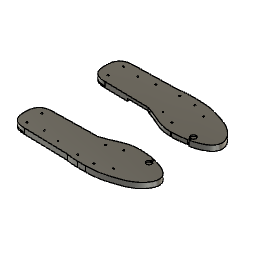
Kids size 4 Insole (Autodesk Fusion 360 design; units mm, degrees)
Autodesk Fusion 360 part; units mm, degrees
note: some values were not read from the file. Chosen so that the rebuilt part matches the saved one: which face or edge a step refers to. Set by a fixed rule: which sketch regions a step uses.
sketch "Sketch2" plane through (0, 0, 0) normal (0, 0, 1) x (1, 0, 0)
  line L0 (0, 0) -> (131.459, 3.2843)
  line L1 (131.459, 3.2843) -> (0, 0.1)
  line L2 (0, 0.1) -> (0, -63.4)
  line L3 (131.459, 3.2843) -> (131.459, -65.9157)
  line L4 (0, -63.4) -> (131.459, -65.9157)
  dimension "d12" = 131.5
  dimension "d13" = 63.5
  dimension "d14" = 69.2
  constraint coincident L0.start origin
  constraint vertical L2
  constraint vertical L3
  measures "d12" distance of L0.start L0.end
  measures "d13" distance of L1.end L2.end
  measures "d14" distance of L0.end L3.end
extrude "Extrude3" add sketch "Sketch2" along normal blind 3 contours L0 L2 L3 L4 makes body 1
fillet "Fillet2" radius 32 tangency weight 1.5916 2 edges at (0, -63.4, 1.5) (0, 0, 1.5) on bodies 1
sketch "Sketch6" plane through (0, 0, 0) normal (0, 0, 1) x (1, 0, 0)
  spline S0 degree 3 poles (0, -31.2105) (0, -25.0639) (0.6991, -19.9859) (3.1095, -12.9138) (4.5302, -10.2219) (8.3444, -5.8662) (10.468, -4.27) (15.3454, -1.7622) (18.03, -0.9116) (24.1411, 0.3806) (27.7349, 0.6929) (31.2008, 0.7795) knots 0 0 0 0 1.843982 1.843982 3.131886 3.131886 4.266621 4.266621 5.428345 5.428345 6.887146 6.887146 6.887146 6.887146
  line L0 (0, -31.2105) -> (0, -32.0065)
  spline S1 degree 3 poles (31.3877, -64.0007) (25.2343, -63.8829) (20.16, -63.0847) (13.1213, -60.5347) (10.451, -59.0604) (6.1653, -55.1613) (4.61, -53.0089) (2.1872, -48.0616) (1.3883, -45.3347) (0.2265, -39.1397) (0, -35.5051) (0, -32.0065) knots 0 0 0 0 1.846381 1.846381 3.135313 3.135313 4.268701 4.268701 5.439843 5.439843 6.910617 6.910617 6.910617 6.910617
  line L1 (31.3877, -64.0007) -> (131.459, -65.9157)
  line L2 (131.459, -65.9157) -> (131.459, 3.2843)
  line L3 (131.459, 3.2843) -> (31.2008, 0.7795)
sketch "Sketch7" plane through (0, 0, 0) normal (0, 0, 1) x (1, 0, 0)
  line L0 (131.459, 3.2843) -> (156.459, 3.2906)
  line L1 (156.459, 3.2906) -> (156.4583, 5.7906)
  line L2 (156.4583, 5.7906) -> (181.4583, 5.7969)
  line L3 (181.4583, 5.7969) -> (206.4583, 5.8032)
  line L4 (206.4583, 5.8032) -> (206.4591, 2.8032)
  line L5 (206.4591, 2.8032) -> (231.4591, 2.8095)
  line L6 (231.4591, 2.8095) -> (231.4609, -4.1905)
  line L7 (231.4609, -4.1905) -> (256.4609, -4.1842)
  line L8 (256.4609, -4.1842) -> (256.4634, -14.1842)
  line L9 (256.4634, -14.1842) -> (281.4634, -14.1779)
  line L10 (281.4634, -14.1779) -> (281.4697, -39.1779)
  line L11 (281.4697, -39.1779) -> (282.4697, -39.1777)
  line L12 (282.4697, -39.1777) -> (282.4728, -51.6776)
  line L13 (282.4728, -51.6776) -> (282.476, -64.1776)
  line L14 (282.476, -64.1776) -> (281.476, -64.1779)
  line L15 (281.476, -64.1779) -> (281.481, -84.1779)
  line L16 (281.481, -84.1779) -> (241.481, -84.188)
  line L17 (241.481, -84.188) -> (241.482, -88.188)
  line L18 (241.482, -88.188) -> (206.482, -88.1968)
  line L19 (206.482, -88.1968) -> (181.482, -88.2031)
  line L20 (181.482, -88.2031) -> (181.4813, -85.2031)
  line L21 (181.4813, -85.2031) -> (156.4813, -85.2094)
  line L22 (156.4813, -85.2094) -> (156.4787, -75.2094)
  line L23 (156.4787, -75.2094) -> (131.4787, -75.2157)
  spline S0 degree 5 poles (131.459, 3.2843) (132.1496, 3.4582) (133.6274, 3.7925) (136.1339, 4.2533) (140.0557, 4.7865) (145.907, 5.3153) (152.6506, 5.6995) (160.1734, 5.9262) (168.2781, 5.9729) (176.6933, 5.8104) (185.1183, 5.4099) (193.2584, 4.7498) (200.8653, 3.8224) (207.7726, 2.6398) (213.9395, 1.2425) (219.4754, -0.2985) (224.5797, -1.9091) (229.489, -3.5365) (234.4262, -5.1721) (239.5391, -6.8834) (244.8868, -8.8023) (250.4574, -11.0844) (256.1762, -13.8773) (261.9178, -17.2853) (267.5158, -21.3344) (272.7732, -25.9844) (277.4708, -31.1438) (281.3773, -36.6842) (284.2586, -42.4544) (285.885, -48.2944) (286.0533, -54.0471) (284.622, -59.5649) (281.5417, -64.7188) (276.8896, -69.4065) (270.8971, -73.5598) (263.8956, -77.1412) (256.2691, -80.1407) (248.4036, -82.5733) (240.6395, -84.4754) (233.2193, -85.9023) (226.2451, -86.925) (219.7173, -87.6165) (213.567, -88.0406) (207.6915, -88.2384) (201.9861, -88.2175) (196.3828, -87.9356) (190.8475, -87.3214) (185.3659, -86.3069) (179.934, -84.8529) (174.5451, -82.9834) (169.1831, -80.7989) (163.8289, -78.4374) (158.4649, -76.0438) (153.0796, -73.7396) (147.6736, -71.5841) (142.2576, -69.5788) (137.9285, -68.0722) (134.6896, -66.981) (132.5348, -66.2682) (131.4585, -65.9154) knots 0 0 0 0 0 0 0.018182 0.036364 0.054545 0.072727 0.090909 0.109091 0.127273 0.145455 0.163636 0.181818 0.2 0.218182 0.236364 0.254545 0.272727 0.290909 0.309091 0.327273 0.345455 0.363636 0.381818 0.4 0.418182 0.436364 0.454545 0.472727 0.490909 0.509091 0.527273 0.545455 0.563636 0.581818 0.6 0.618182 0.636364 0.654545 0.672727 0.690909 0.709091 0.727273 0.745455 0.763636 0.781818 0.8 0.818182 0.836364 0.854545 0.872727 0.890909 0.909091 0.927273 0.945455 0.963636 0.981818 1 1 1 1 1 1
  line L24 (131.459, 3.2843) -> (131.4585, -65.9154)
  line L25 (152.0683, -72.6702) -> (110.8487, -59.1606)
  point P0 (131.459, 3.2843)
  dimension "d41" = 25
  dimension "d42" = 2.5
  dimension "d43" = 25
  dimension "d44" = 25
  dimension "d45" = 3
  dimension "d46" = 25
  dimension "d47" = 7
  dimension "d48" = 25
  dimension "d49" = 10
  dimension "d50" = 25
  dimension "d51" = 25
  dimension "d52" = 1
  dimension "d53" = 12.5
  dimension "d54" = 12.5
  dimension "d55" = 1
  dimension "d56" = 20
  dimension "d57" = 40
  dimension "d58" = 4
  dimension "d59" = 35
  dimension "d60" = 25
  dimension "d63" = 3
  dimension "d64" = 25
  dimension "d65" = 10
  dimension "d66" = 25
  constraint coincident P0 L0.start
  constraint perpendicular L0 L1
  constraint perpendicular L1 L2
  constraint parallel L2 L3
  constraint perpendicular L3 L4
  constraint perpendicular L4 L5
  constraint perpendicular L5 L6
  constraint perpendicular L6 L7
  constraint perpendicular L7 L8
  constraint perpendicular L8 L9
  constraint perpendicular L9 L10
  constraint perpendicular L10 L11
  constraint perpendicular L11 L12
  constraint parallel L12 L13
  constraint perpendicular L13 L14
  constraint perpendicular L14 L15
  constraint perpendicular L15 L16
  constraint perpendicular L16 L17
  constraint perpendicular L17 L18
  constraint parallel L18 L19
  constraint perpendicular L19 L20
  constraint perpendicular L20 L21
  constraint perpendicular L21 L22
  constraint perpendicular L22 L23
  constraint midpoint S0.end L25
  measures "d41" distance of P0 L0.end
  measures "d42" distance of L0.end L1.end
  measures "d43" distance of L1.end L2.end
  measures "d44" distance of L2.end L3.end
  measures "d45" distance of L3.end L4.end
  measures "d46" distance of L4.end L5.end
  measures "d47" distance of L5.end L6.end
  measures "d48" distance of L6.end L7.end
  measures "d49" distance of L7.end L8.end
  measures "d50" distance of L8.end L9.end
  measures "d51" distance of L9.end L10.end
  measures "d52" distance of L10.end L11.end
  measures "d53" distance of L11.end L12.end
  measures "d54" distance of L12.end L13.end
  measures "d55" distance of L13.end L14.end
  measures "d56" distance of L14.end L15.end
  measures "d57" distance of L15.end L16.end
  measures "d58" distance of L16.end L17.end
  measures "d59" distance of L17.end L18.end
  measures "d60" distance of L18.end L19.end
  measures "d63" distance of L19.end L20.end
  measures "d64" distance of L20.end L21.end
  measures "d65" distance of L21.end L22.end
  measures "d66" distance of L22.end L23.end
extrude "Extrude5" add sketch "Sketch7" along normal blind 3 contours L0 L1 S0 | L0 L1 L2 L10 L11 L12 L13 L19 S0 L24 | L10 L11 S0 | L12 L13 S0 bodies 1
hole "Hole2" at (144.8302, -7.2652, 3) direction (0, 0, -1) diameter 3.66 depth 25 tip angle 118 bodies 1
hole "Hole3" at (157.2563, -58.0502, 3) direction (0, 0, -1) diameter 3.66 depth 25 tip angle 118 bodies 1
hole "Hole4" at (23.0004, -13.2082, 3) direction (0, 0, -1) diameter 3.66 depth 25 tip angle 118 bodies 1
hole "Hole5" at (22.3251, -47.9202, 3) direction (0, 0, -1) diameter 3.66 depth 25 tip angle 118 bodies 1
hole "Hole6" at (94.9908, -11.9926, 3) direction (0, 0, -1) diameter 3.66 depth 25 tip angle 118 bodies 1
extrude "Extrude6" add 1 faces at (85.7573, -47.8831, 3) along direction (0, 0, 1) blind 9.25 on bodies 1 bodies 1
hole "Hole8" at (180.2887, -8.2307, 12.25) direction (0, 0, -1) diameter 3.66 depth 25 tip angle 118 bodies 1
hole "Hole9" at (58.9598, -17.4028, 12.25) direction (0, 0, -1) diameter 3.66 depth 25 tip angle 118 bodies 1
hole "Hole10" at (212.5454, -20.8108, 12.25) direction (0, 0, -1) diameter 3.66 depth 25 tip angle 118 bodies 1
hole "Hole12" at (188.1637, -68.6508, 0) direction (0, 0, 1) diameter 3.66 depth 15 tip angle 118 bodies 1
hole "Hole7" at (241.4162, -72.7282, 12.25) direction (0, 0, -1) diameter 12.2 depth 3 tip angle 180 bodies 1
sketch "Sketch8" plane through (0, 0, 12.25) normal (0, 0, 1) x (1, 0, 0)
  line L0 (242.7662, -72.7282) -> (240.0662, -72.7282)
  line L1 (240.0662, -72.7282) -> (240.0662, -84.5002)
  line L2 (240.0662, -84.5002) -> (242.7662, -84.5002)
  line L3 (242.7662, -84.5002) -> (242.7662, -72.7282)
  circle A0 centre (94.9908, -11.9926) radius 1.83
  circle A1 centre (22.3251, -47.9202) radius 1.83
  circle A2 centre (23.0004, -13.2082) radius 1.83
  circle A3 centre (157.2563, -58.0502) radius 1.83
  circle A4 centre (144.8302, -7.2652) radius 1.83
  spline S0 degree 3 poles (31.2008, 0.7795) (27.7349, 0.6929) (24.1411, 0.3806) (18.03, -0.9116) (15.3454, -1.7622) (10.468, -4.27) (8.3444, -5.8662) (4.5302, -10.2219) (3.1095, -12.9138) (0.6991, -19.9859) (0, -25.0639) (0, -31.2105) knots -6.887146 -6.887146 -6.887146 -6.887146 -5.428345 -5.428345 -4.266621 -4.266621 -3.131886 -3.131886 -1.843982 -1.843982 0 0 0 0
  line L4 (0, -31.2105) -> (0, -32.0065)
  spline S1 degree 3 poles (0, -32.0065) (0, -35.5051) (0.2265, -39.1397) (1.3883, -45.3347) (2.1872, -48.0616) (4.61, -53.0089) (6.1653, -55.1613) (10.451, -59.0604) (13.1213, -60.5347) (20.16, -63.0847) (25.2343, -63.8829) (31.3877, -64.0007) knots -6.910617 -6.910617 -6.910617 -6.910617 -5.439843 -5.439843 -4.268701 -4.268701 -3.135313 -3.135313 -1.846381 -1.846381 0 0 0 0
  line L5 (31.3877, -64.0007) -> (131.459, -65.9157)
  spline S2 degree 5 poles (131.459, -65.9156) (132.5352, -66.2683) (134.6899, -66.9811) (137.9287, -68.0722) (142.2577, -69.5788) (147.6736, -71.5841) (153.0796, -73.7396) (158.4649, -76.0438) (163.8289, -78.4374) (169.1831, -80.7989) (174.5451, -82.9834) (179.934, -84.8529) (185.3659, -86.3069) (190.8475, -87.3214) (195.8051, -87.8715) (199.6969, -88.0977) (202.4992, -88.175) (204.1845, -88.1939) (204.7313, -88.1972) knots -0.999998 -0.999998 -0.999998 -0.999998 -0.999998 -0.999998 -0.981818 -0.963636 -0.945455 -0.927273 -0.909091 -0.890909 -0.872727 -0.854545 -0.836364 -0.818182 -0.8 -0.781818 -0.763636 -0.754941 -0.754941 -0.754941 -0.754941 -0.754941 -0.754941
  line L6 (204.7313, -88.1972) -> (206.482, -88.1968)
  spline S3 degree 5 poles (206.482, -88.1968) (206.7317, -88.1952) (208.1358, -88.183) (210.716, -88.1299) (214.5305, -87.9742) (219.7173, -87.6165) (226.2451, -86.925) (233.2193, -85.9023) (240.6395, -84.4754) (248.4036, -82.5733) (256.2691, -80.1407) (263.8956, -77.1412) (270.8971, -73.5598) (276.8896, -69.4065) (281.5417, -64.7188) (284.622, -59.5649) (286.0533, -54.0471) (285.885, -48.2944) (284.2586, -42.4544) (281.3773, -36.6842) (277.4708, -31.1438) (272.7732, -25.9844) (267.5158, -21.3344) (261.9178, -17.2853) (256.1762, -13.8773) (250.4574, -11.0844) (244.8868, -8.8023) (239.5391, -6.8834) (234.4262, -5.1721) (229.489, -3.5365) (224.5797, -1.9091) (219.4754, -0.2985) (213.9395, 1.2425) (207.7726, 2.6398) (200.8653, 3.8224) (193.2584, 4.7498) (186.4723, 5.3001) (181.1712, 5.5881) (177.5263, 5.7278) (175.5655, 5.7871) (175.283, 5.7954) knots -0.749394 -0.749394 -0.749394 -0.749394 -0.749394 -0.749394 -0.745455 -0.727273 -0.709091 -0.690909 -0.672727 -0.654545 -0.636364 -0.618182 -0.6 -0.581818 -0.563636 -0.545455 -0.527273 -0.509091 -0.490909 -0.472727 -0.454545 -0.436364 -0.418182 -0.4 -0.381818 -0.363636 -0.345455 -0.327273 -0.309091 -0.290909 -0.272727 -0.254545 -0.236364 -0.218182 -0.2 -0.181818 -0.163636 -0.145455 -0.127273 -0.124212 -0.124212 -0.124212 -0.124212 -0.124212 -0.124212
  line L7 (175.283, 5.7954) -> (156.4583, 5.7906)
  spline S4 degree 5 poles (156.4583, 5.7906) (155.7183, 5.7686) (153.5076, 5.6957) (149.9506, 5.5432) (145.3158, 5.2618) (140.0557, 4.7865) (136.1339, 4.2533) (133.6274, 3.7925) (132.1496, 3.4582) (131.459, 3.2843) knots -0.081724 -0.081724 -0.081724 -0.081724 -0.081724 -0.081724 -0.072727 -0.054545 -0.036364 -0.018182 0 0 0 0 0 0
  line L8 (131.459, 3.2843) -> (31.2008, 0.7795)
  circle A5 centre (212.5454, -20.8108) radius 1.83
  circle A6 centre (58.9598, -17.4028) radius 1.83
  circle A7 centre (180.2887, -8.2307) radius 1.83
  circle A8 centre (188.1637, -68.6508) radius 1.83
  circle A9 centre (241.4162, -72.7282) radius 6.1
  point P0 (241.4162, -72.7282)
  point P1 (241.4162, -72.7282)
  point P2 (241.4162, -72.7282)
  dimension "d91" = 2.7
  constraint horizontal L0
  constraint vertical L1
  constraint horizontal L2
  constraint vertical L3
  constraint midpoint L0 P2
  constraint coincident P2 P1
  constraint coincident L1.end S3
  measures "d91" distance of L0.start L0.end
extrude "Extrude7" cut sketch "Sketch8" against normal blind 2.7 contours L1 L3 S3 A9 bodies 1
sketch "Sketch9" plane through (0, 0, 0) normal (0, 0, 1) x (1, 0, 0)
  line L0 (83.1727, -66.3805) -> (151.6727, -66.3805)
  line L1 (151.6727, -66.3805) -> (151.6727, -18.3805)
  line L2 (151.6727, -18.3805) -> (83.1727, -18.3805)
  line L3 (83.1727, -18.3805) -> (83.1727, -66.3805)
  dimension "d94" = 68.5
  dimension "d214" = 48
  constraint horizontal L0
  constraint vertical L1
  constraint horizontal L2
  constraint vertical L3
  measures "d94" distance of L0.start L0.end
  measures "d214" distance of L0.start L2.end
extrude "Extrude8" cut sketch "Sketch9" along normal blind 5.5 bodies 1
sketch "Sketch21" plane through (0, 0, 0) normal (0, 0, -1) x (1, 0, 0)
  line L0 (83.1727, 18.3805) -> (83.1727, 64.9916)
  line L1 (83.1727, 64.9916) -> (31.3877, 64.0007)
  spline S0 degree 3 poles (0, 32.0065) (0, 38.1611) (0.7009, 43.2497) (3.1158, 50.3359) (4.5388, 53.034) (8.3551, 57.3935) (10.4774, 58.9897) (15.3774, 61.5066) (18.0886, 62.3576) (24.2602, 63.6377) (27.8898, 63.9337) (31.3877, 64.0007) knots 0 0 0 0 1.846381 1.846381 3.135313 3.135313 4.268701 4.268701 5.439843 5.439843 6.910617 6.910617 6.910617 6.910617
  line L2 (0, 32.0065) -> (0, 31.2105)
  spline S1 degree 3 poles (31.2008, -0.7795) (25.0561, -0.626) (19.9971, 0.1997) (12.9875, 2.786) (10.3318, 4.2735) (6.0727, 8.1953) (4.5301, 10.3581) (2.1449, 15.2966) (1.3617, 18.0016) (0.2224, 24.1431) (0, 27.7435) (0, 31.2105) knots 0 0 0 0 1.843982 1.843982 3.131886 3.131886 4.266621 4.266621 5.428345 5.428345 6.887146 6.887146 6.887146 6.887146
  line L3 (31.2008, -0.7795) -> (131.459, -3.2843)
  spline S2 degree 5 poles (131.459, -3.2843) (132.1496, -3.4582) (133.6274, -3.7925) (136.1339, -4.2533) (140.0557, -4.7865) (145.3158, -5.2618) (149.9506, -5.5432) (153.5076, -5.6957) (155.7183, -5.7686) (156.4583, -5.7906) knots 0 0 0 0 0 0 0.018182 0.036364 0.054545 0.072727 0.081724 0.081724 0.081724 0.081724 0.081724 0.081724
  line L4 (156.4583, -5.7906) -> (175.283, -5.7954)
  spline S3 degree 5 poles (175.283, -5.7954) (175.5655, -5.7871) (177.5263, -5.7278) (181.1712, -5.5881) (186.4723, -5.3001) (193.2584, -4.7498) (200.8653, -3.8224) (207.7726, -2.6398) (213.9395, -1.2425) (219.4754, 0.2985) (224.5797, 1.9091) (229.489, 3.5365) (234.4262, 5.1721) (239.5391, 6.8834) (244.8868, 8.8023) (250.4574, 11.0844) (256.1762, 13.8773) (261.9178, 17.2853) (267.5158, 21.3344) (272.7732, 25.9844) (277.4708, 31.1438) (281.3773, 36.6842) (284.2586, 42.4544) (285.885, 48.2944) (286.0533, 54.0471) (284.622, 59.5649) (281.5417, 64.7188) (276.8896, 69.4065) (270.8971, 73.5598) (263.8956, 77.1412) (256.2691, 80.1407) (248.4036, 82.5733) (240.6395, 84.4754) (233.2193, 85.9023) (226.2451, 86.925) (219.7173, 87.6165) (214.5305, 87.9742) (210.716, 88.1299) (208.1358, 88.183) (206.7317, 88.1952) (206.482, 88.1968) knots 0.124212 0.124212 0.124212 0.124212 0.124212 0.124212 0.127273 0.145455 0.163636 0.181818 0.2 0.218182 0.236364 0.254545 0.272727 0.290909 0.309091 0.327273 0.345455 0.363636 0.381818 0.4 0.418182 0.436364 0.454545 0.472727 0.490909 0.509091 0.527273 0.545455 0.563636 0.581818 0.6 0.618182 0.636364 0.654545 0.672727 0.690909 0.709091 0.727273 0.745455 0.749394 0.749394 0.749394 0.749394 0.749394 0.749394
  line L5 (206.482, 88.1968) -> (204.7313, 88.1972)
  spline S4 degree 5 poles (204.7313, 88.1972) (204.1845, 88.1939) (202.4992, 88.175) (199.6969, 88.0977) (195.8051, 87.8715) (190.8475, 87.3214) (185.3659, 86.3069) (179.934, 84.8529) (174.5451, 82.9834) (169.1831, 80.7989) (163.8289, 78.4374) (158.4649, 76.0438) (153.0796, 73.7396) (147.6736, 71.5841) (142.5416, 69.684) (138.4961, 68.2701) (135.5392, 67.2681) (133.6655, 66.6436) (132.8706, 66.3805) knots 0.754941 0.754941 0.754941 0.754941 0.754941 0.754941 0.763636 0.781818 0.8 0.818182 0.836364 0.854545 0.872727 0.890909 0.909091 0.927273 0.945455 0.963636 0.981818 0.995232 0.995232 0.995232 0.995232 0.995232 0.995232
  line L6 (151.6727, 66.3805) -> (151.6727, 18.3805)
  line L7 (151.6727, 18.3805) -> (83.1727, 18.3805)
  circle A0 centre (212.5454, 20.8108) radius 1.83
  circle A1 centre (180.2887, 8.2307) radius 1.83
  circle A2 centre (94.9908, 11.9926) radius 1.83
  circle A3 centre (22.3251, 47.9202) radius 1.83
  circle A4 centre (23.0004, 13.2082) radius 1.83
  circle A5 centre (157.2563, 58.0502) radius 1.83
  circle A6 centre (144.8302, 7.2652) radius 1.83
  spline S5 degree 3 poles (174.4959, -3.7952) (181.2263, -3.8053) (187.9966, -3.5849) (194.1763, -3.0866) (199.6761, -2.6431) (204.6893, -1.9777) (209.1349, -1.1477) (216.1409, 0.1603) (221.7765, 1.8345) (227.4131, 3.5051) (231.588, 4.7425) (235.7978, 5.9662) (240.2462, 7.4095) (245.0183, 8.9579) (250.063, 10.8078) (255.1618, 13.3897) (259.9992, 15.8392) (264.8777, 18.9635) (269.2794, 22.7035) (274.7206, 27.3269) (279.4009, 32.8838) (282.1056, 38.5417) (284.1078, 42.7301) (285.0101, 46.9222) (284.5798, 50.872) (284.1825, 54.5194) (282.6528, 58.0122) (279.9084, 61.3117) (277.0673, 64.7275) (272.91, 67.9026) (267.9776, 70.6517) (262.5278, 73.6892) (256.1876, 76.2039) (249.9117, 78.1747) (244.1413, 79.9868) (238.4521, 81.345) (233.1705, 82.3571) (226.4333, 83.6481) (220.3368, 84.3983) (214.6293, 84.8401) (212.5323, 85.0024) (210.483, 85.1211) (208.4645, 85.1963) knots 0.124276 0.124276 0.124276 0.124276 0.168305 0.168305 0.168305 0.20749 0.20749 0.20749 0.269244 0.269244 0.269244 0.314984 0.314984 0.314984 0.364052 0.364052 0.364052 0.410606 0.410606 0.410606 0.468154 0.468154 0.468154 0.510756 0.510756 0.510756 0.550097 0.550097 0.550097 0.590825 0.590825 0.590825 0.635825 0.635825 0.635825 0.677202 0.677202 0.677202 0.729983 0.729983 0.729983 0.749375 0.749375 0.749375 0.749375
  line L8 (208.4645, 85.1963) -> (204.7552, 85.1972)
  spline S6 degree 3 poles (204.7552, 85.1972) (198.4322, 85.2168) (192.3757, 84.7871) (186.3988, 83.5447) (181.5065, 82.5277) (176.67, 80.9335) (171.7851, 78.9909) (166.3832, 76.8426) (160.9144, 74.3395) (155.3757, 72.069) (149.1154, 69.5026) (142.7961, 67.2432) (136.5459, 65.1891) (134.9933, 64.6788) (133.4441, 64.1791) (131.8978, 63.6881) (131.0209, 63.4096) (130.144, 63.1312) (129.2671, 62.8527) knots 0.754962 0.754962 0.754962 0.754962 0.816206 0.816206 0.816206 0.866336 0.866336 0.866336 0.921773 0.921773 0.921773 0.984433 0.984433 0.984433 0.999998 0.999998 0.999998 1.00886 1.00886 1.00886 1.00886
  line L9 (129.459, 63.877) -> (170.4335, 64.6611)
  line L10 (170.4335, 64.6611) -> (170.4335, 14.9026)
  line L11 (170.4335, 14.9026) -> (60.8601, 14.9026)
  arc A7 (54.9736, 19.7546) -> (60.8601, 14.9026) centre (59.2939, 18.9992) ccw
  line L12 (54.9736, 19.7546) -> (28.5352, 19.7546)
  line L13 (28.5352, 19.7546) -> (28.5352, 61.9457)
  line L14 (28.5352, 61.9457) -> (31.426, 62.001)
  spline S7 degree 3 poles (2, 32.0065) (2, 38.0093) (2.6894, 42.8845) (4.0162, 46.7776) (4.9423, 49.4954) (6.2449, 51.9465) (8.0743, 54.0363) (9.6832, 55.8742) (11.5883, 57.3119) (13.8011, 58.4485) (16.0871, 59.6228) (18.6268, 60.4267) (21.2306, 60.9668) (24.4999, 61.6449) (28.0143, 61.9357) (31.426, 62.001) knots 0 0 0 0 1.846381 1.846381 1.846381 3.135313 3.135313 3.135313 4.268701 4.268701 4.268701 5.439843 5.439843 5.439843 6.910617 6.910617 6.910617 6.910617
  line L15 (2, 32.0065) -> (2, 31.2105)
  spline S8 degree 3 poles (31.2507, 1.2199) (25.2576, 1.3696) (20.4117, 2.1785) (16.5623, 3.5988) (13.8737, 4.5908) (11.4621, 5.9515) (9.4224, 7.8296) (7.625, 9.4846) (6.2351, 11.4266) (5.1525, 13.6682) (4.0444, 15.9626) (3.3038, 18.4975) (2.8231, 21.089) (2.2195, 24.3428) (2, 27.8291) (2, 31.2105) knots 0 0 0 0 1.843982 1.843982 1.843982 3.131886 3.131886 3.131886 4.266621 4.266621 4.266621 5.428345 5.428345 5.428345 6.887146 6.887146 6.887146 6.887146
  line L16 (31.2507, 1.2199) -> (131.7315, -1.2905)
  spline S9 degree 3 poles (131.7315, -1.2905) (131.8034, -1.3086) (131.8754, -1.3267) (131.9473, -1.3449) (135.315, -2.1928) (140.3954, -2.88) (146.9368, -3.3312) (149.8544, -3.5324) (153.0601, -3.6881) (156.4884, -3.7906) knots -0.001137 -0.001137 -0.001137 -0.001137 0 0 0 0.056467 0.056467 0.056467 0.081652 0.081652 0.081652 0.081652
  line L17 (156.4884, -3.7906) -> (174.4959, -3.7952)
  line L18 (240.0662, 78.6769) -> (240.0662, 84.5002)
  spline S10 degree 3 poles (242.7662, 83.892) (241.8683, 84.103) (240.9678, 84.3057) (240.0662, 84.5002) knots -0.327778 -0.327778 -0.327778 -0.327778 -0.051126 -0.051126 -0.051126 -0.051126
  line L19 (242.7662, 83.892) -> (242.7662, 78.6769)
  line L20 (170.4335, 64.6611) -> (151.6727, 64.6611)
  line L21 (242.7662, 80.2108) -> (242.7662, 83.892)
  line L22 (129.459, 63.877) -> (132.6851, 63.9388)
  circle A8 centre (188.1637, 68.6508) radius 1.83
  arc A9 (242.7662, 78.6769) -> (240.0662, 78.6769) centre (241.4162, 72.7282) ccw
  line L23 (132.8706, 66.3805) -> (151.6727, 66.3805)
  circle A10 centre (58.9598, 17.4028) radius 1.83
  constraint coincident L6 L20.end
  constraint perpendicular L6 L20
  constraint coincident S5 L21.start
  constraint coincident S10.start L19.start
  constraint parallel L19 L21
  constraint coincident S6 L22.end
  constraint parallel L9 L22
extrude "Extrude23" cut sketch "Sketch21" against normal blind 3 contours S3 L5 S4 S5 L8 S6 L18 L23 bodies 1
extrude "Extrude24" cut sketch "Sketch21" against normal blind 10 contours S3 S5 L18 S10 L19 L21 bodies 1
fillet "Fillet12" radius 3 1 edges at (240.0662, -82.6896, 3) on bodies 1
sketch "Sketch27" plane through (0, 0, 0) normal (0, 0, 1) x (1, 0, 0)
  line L0 (20.4951, -46.4) -> (83.1727, -46.4)
  line L1 (83.1727, -46.4) -> (83.1727, -49.5)
  line L2 (83.1727, -49.5) -> (20.4951, -49.5)
  line L3 (20.4951, -49.5) -> (20.4951, -46.4)
  line L4 (30.3437, -19.2975) -> (27.7144, -21.5186)
  line L5 (27.7144, -21.5186) -> (21.5988, -14.2792)
  line L6 (21.5988, -14.2792) -> (24.2282, -12.058)
  line L7 (24.2282, -12.058) -> (30.3437, -19.2975)
  line L8 (96.5, -12) -> (93.5, -12)
  line L9 (93.5, -12) -> (93.5, -21.9489)
  line L10 (93.5, -21.9489) -> (96.5, -21.9489)
  line L11 (96.5, -21.9489) -> (96.5, -12)
  line L12 (212.5, -19.2931) -> (143.1326, -19.2931)
  line L13 (143.1326, -19.2931) -> (143.1326, -22.7134)
  line L14 (143.1326, -22.7134) -> (212.5, -22.7134)
  line L15 (212.5, -22.7134) -> (212.5, -19.2931)
  line L16 (146.358, -7.2179) -> (143.1326, -7.2179)
  line L17 (143.1326, -7.2179) -> (143.1326, -22.7134)
  line L18 (143.1326, -22.7134) -> (146.358, -22.7134)
  line L19 (146.358, -22.7134) -> (146.358, -7.2179)
  line L20 (181.8156, -8.2316) -> (178.7964, -8.2316)
  line L21 (178.7964, -8.2316) -> (178.7964, -22.7134)
  line L22 (178.7964, -22.7134) -> (181.8156, -22.7134)
  line L23 (181.8156, -22.7134) -> (181.8156, -8.2316)
  line L24 (189, -67.5) -> (155.8814, -55.4458)
  line L25 (155.8814, -55.4458) -> (154.7108, -58.662)
  line L26 (154.7108, -58.662) -> (187.8294, -70.7162)
  line L27 (187.8294, -70.7162) -> (189, -67.5)
  line L28 (83.1727, -18.3805) -> (83.1727, -64.9916)
  line L29 (83.1727, -18.3805) -> (27.4949, -18.3805)
  line L30 (27.4949, -18.3805) -> (27.4949, -21.4805)
  line L31 (27.4949, -21.4805) -> (83.1727, -21.4805)
  line L32 (83.1727, -21.4805) -> (83.1727, -18.3805)
  line L33 (157.2563, -56.2202) -> (151.6727, -56.2202)
  line L34 (151.6727, -56.2202) -> (151.6727, -59.0451)
  line L35 (151.6727, -59.0451) -> (157.2563, -59.0451)
  line L36 (157.2563, -59.0451) -> (157.2563, -56.2202)
  circle A0 centre (157.2563, -58.0502) radius 1.83
  line L37 (151.6727, -66.3805) -> (151.6727, -18.3805)
  point P0 (20.4951, -47.9202)
  dimension "d190" = 3
  dimension "d215" = 3.1
  dimension "d216" = 3.1
  constraint horizontal L0
  constraint vertical L1
  constraint horizontal L2
  constraint vertical L3
  constraint perpendicular L4 L5
  constraint parallel L4 L6
  constraint parallel L5 L7
  constraint horizontal L8
  constraint vertical L9
  constraint horizontal L10
  constraint vertical L11
  constraint horizontal L12
  constraint vertical L13
  constraint horizontal L14
  constraint vertical L15
  constraint horizontal L16
  constraint vertical L17
  constraint horizontal L18
  constraint vertical L19
  constraint coincident L14 L13.end
  constraint horizontal L20
  constraint vertical L21
  constraint horizontal L22
  constraint vertical L23
  constraint coincident L14 L21.end
  constraint perpendicular L24 L25
  constraint parallel L24 L26
  constraint parallel L25 L27
  constraint coincident L12.end L17
  constraint coincident L3 P0
  constraint coincident L0.end L28
  constraint horizontal L29
  constraint vertical L30
  constraint horizontal L31
  constraint vertical L32
  constraint coincident L28.start L29.start
  constraint horizontal L33
  constraint vertical L34
  constraint horizontal L35
  constraint vertical L36
  constraint coincident L33.start A0
  constraint coincident L33.end L37
  measures "d190" distance of L8.start L8.end
  measures "d215" distance of L0.end L1.end
  measures "d216" distance of L28.start L31.end
extrude "Extrude30" cut sketch "Sketch27" along normal blind 1 contours L0 L1 L2 L3 L28 | L4 L7 L28 L29 L31 L32 | L4 L5 L7 L29 L30 L31 | L4 L5 L31 | L5 L6 L7 L29 L30 | L8 L9 L10 L11 | L12 L14 L15 L23 | L12 L14 L21 L22 L23 | L12 L20 L21 L23 | L12 L14 L21 L37 | L12 L14 L19 L37 | L12 L13 L14 L17 L18 L19 | L12 L16 L17 L19 | L24 L25 L26 L27 L33 A0 | L25 L26 L33 A0 | L25 L26 L33 L34 L35 A0 L37 | L26 L35 L36 A0 | L26 L35 L36 A0 bodies 1
extrude "Extrude31" cut sketch "Sketch27" along normal blind 2 contours L12 L14 L21 L37 | L12 L14 L19 L37 | L12 L13 L14 L17 L18 L19 | L25 L26 L33 L34 L35 A0 L37 bodies 1
ref_plane "WorkPlane1" through (0, -100, 0) normal (0, 1, 0) x (0, 0, 1)
scale "Scale1" factor 0.82 about (175.283, 5.7954, 12.25) bodies 1
mirror "Mirror1" about plane through (0, -100, 0) normal (0, 1, 0) of bodies 1 makes body 2
sketch "Sketch29" plane through (0, 0, 12.25) normal (0, 0, 1) x (-1, 0, 0)
  circle A0 centre (-150.3117, 4.9143) radius 1.5006
  circle A1 centre (-160.5011, 46.558) radius 1.5006
  circle A2 centre (-50.4113, 9.7875) radius 1.5006
  circle A3 centre (-49.8575, 38.2514) radius 1.5006
  circle A4 centre (-109.4434, 8.7907) radius 1.5006
  circle A5 centre (-179.3877, 5.706) radius 1.5006
  circle A6 centre (-79.898, 13.2271) radius 1.5006
  circle A7 centre (-205.8382, 16.0217) radius 1.5006
  circle A8 centre (-185.8451, 55.2505) radius 1.5006
  line L0 (-228.4052, 68.247) -> (-228.4052, 63.4719)
  arc A9 (-230.6192, 63.4719) -> (-228.4052, 63.4719) centre (-229.5122, 58.594) ccw
  line L1 (-230.6192, 63.4719) -> (-230.6192, 67.7483)
  spline S0 degree 5 poles (-230.6192, 67.7483) (-231.5384, 67.5324) (-233.7274, 66.9961) (-237.2226, 66.0525) (-242.0268, 64.5404) (-247.9454, 62.2126) (-253.6866, 59.2759) (-258.6005, 55.8702) (-262.4151, 52.0263) (-264.941, 47.8) (-266.1146, 43.2754) (-265.9766, 38.5583) (-264.643, 33.7694) (-262.2803, 29.0379) (-259.077, 24.4947) (-255.2249, 20.264) (-250.9139, 16.4511) (-246.3235, 13.1308) (-241.6155, 10.3362) (-236.926, 8.046) (-232.3581, 6.1747) (-227.973, 4.6012) (-223.7804, 3.198) (-219.7319, 1.8568) (-215.7063, 0.5223) (-211.5208, -0.7984) (-206.9813, -2.062) (-201.9245, -3.2078) (-196.2605, -4.1775) (-190.0229, -4.938) (-184.4582, -5.3893) (-180.1113, -5.6254) (-177.1226, -5.74) (-175.5146, -5.7886) (-175.283, -5.7954) knots -0.649672 -0.649672 -0.649672 -0.649672 -0.649672 -0.649672 -0.636364 -0.618182 -0.6 -0.581818 -0.563636 -0.545455 -0.527273 -0.509091 -0.490909 -0.472727 -0.454545 -0.436364 -0.418182 -0.4 -0.381818 -0.363636 -0.345455 -0.327273 -0.309091 -0.290909 -0.272727 -0.254545 -0.236364 -0.218182 -0.2 -0.181818 -0.163636 -0.145455 -0.127273 -0.124212 -0.124212 -0.124212 -0.124212 -0.124212 -0.124212
  line L2 (-175.283, -5.7954) -> (-159.8468, -5.7915)
  spline S1 degree 5 poles (-159.8468, -5.7915) (-159.2399, -5.7734) (-157.4272, -5.7136) (-154.5105, -5.5886) (-150.7099, -5.3579) (-146.3966, -4.9681) (-143.1807, -4.5308) (-141.1254, -4.153) (-139.9136, -3.8789) (-139.3473, -3.7363) knots -0.081724 -0.081724 -0.081724 -0.081724 -0.081724 -0.081724 -0.072727 -0.054545 -0.036364 -0.018182 0 0 0 0 0 0
  line L3 (-139.3473, -3.7363) -> (-57.1356, -1.6824)
  spline S2 degree 3 poles (-57.1356, -1.6824) (-54.2935, -1.6114) (-51.3467, -1.3553) (-46.3356, -0.2956) (-44.1342, 0.4019) (-40.1347, 2.4583) (-38.3933, 3.7671) (-35.2657, 7.3388) (-34.1007, 9.5462) (-32.1242, 15.3453) (-31.5509, 19.5092) (-31.5509, 24.5495) knots -6.887146 -6.887146 -6.887146 -6.887146 -5.428345 -5.428345 -4.266621 -4.266621 -3.131886 -3.131886 -1.843982 -1.843982 0 0 0 0
  line L4 (-31.5509, 24.5495) -> (-31.5509, 25.2022)
  spline S3 degree 3 poles (-31.5509, 25.2022) (-31.5509, 28.0711) (-31.7367, 31.0514) (-32.6893, 36.1313) (-33.3445, 38.3674) (-35.3311, 42.4241) (-36.6065, 44.1891) (-40.1207, 47.3863) (-42.3104, 48.5953) (-48.0822, 50.6863) (-52.243, 51.3408) (-57.2889, 51.4374) knots -6.910617 -6.910617 -6.910617 -6.910617 -5.439843 -5.439843 -4.268701 -4.268701 -3.135313 -3.135313 -1.846381 -1.846381 0 0 0 0
  line L5 (-57.2889, 51.4374) -> (-139.3473, 53.0077)
  line L6 (-139.3473, 53.0077) -> (-139.3473, 53.0076)
  spline S4 degree 5 poles (-139.3473, 53.0076) (-140.2298, 53.2968) (-141.9967, 53.8813) (-144.6524, 54.7761) (-148.2022, 56.0115) (-152.6433, 57.6558) (-157.0762, 59.4233) (-161.4922, 61.3127) (-165.8906, 63.2755) (-170.2811, 65.212) (-174.6779, 67.0032) (-179.0969, 68.5362) (-183.551, 69.7285) (-188.0459, 70.5604) (-192.1112, 71.0115) (-195.3024, 71.197) (-197.6003, 71.2603) (-198.9822, 71.2758) (-199.4306, 71.2786) knots -0.999998 -0.999998 -0.999998 -0.999998 -0.999998 -0.999998 -0.981818 -0.963636 -0.945455 -0.927273 -0.909091 -0.890909 -0.872727 -0.854545 -0.836364 -0.818182 -0.8 -0.781818 -0.763636 -0.754941 -0.754941 -0.754941 -0.754941 -0.754941 -0.754941
  line L7 (-199.4306, 71.2786) -> (-200.8662, 71.2782)
  spline S5 degree 5 poles (-200.8662, 71.2782) (-201.0709, 71.2769) (-202.2223, 71.2669) (-204.338, 71.2234) (-207.466, 71.0957) (-211.7191, 70.8024) (-216.9788, 70.2452) (-221.4481, 69.5935) (-224.9304, 68.9685) (-227.2749, 68.4909) (-228.4052, 68.247) knots -0.749394 -0.749394 -0.749394 -0.749394 -0.749394 -0.749394 -0.745455 -0.727273 -0.709091 -0.690909 -0.672727 -0.656127 -0.656127 -0.656127 -0.656127 -0.656127 -0.656127
  point P0 (-265.6767, 38.531)
  constraint coincident S0 P0
